Autodesk Inventor part; units mm, degrees
(part 4 of 18)
  ellipse E454 centre (-10072.3071, -10029.7963) end of major axis (-10072.1176, -10029.8098) minor radius 0.0836 (-10072.3568, -10029.8743) -> (-10072.2798, -10029.8808) ccw
  ellipse E455 centre (-10072.3658, -10028.6299) end of major axis (-10072.5466, -10028.6883) minor radius 0.168 (-10072.5392, -10028.5756) -> (-10072.5534, -10028.6311) ccw
  ellipse E456 centre (-10070.2632, -10029.6485) end of major axis (-10070.4527, -10029.6349) minor radius 0.0836 (-10070.2359, -10029.733) -> (-10070.1721, -10029.7273) ccw
  ellipse E457 centre (-10072.2975, -10029.6619) end of major axis (-10072.487, -10029.6483) minor radius 0.0836 (-10072.3473, -10029.7399) -> (-10072.2702, -10029.7464) ccw
  line L566 (-10072.7988, -10029.4384) -> (-10074.1814, -10029.4475)
  line L567 (-10074.3417, -10029.5333) -> (-10074.2688, -10029.759)
  line L568 (-10068.3003, -10029.8537) -> (-10068.4165, -10029.4942)
  line L569 (-10068.6314, -10029.4109) -> (-10070.0139, -10029.4201)
  line L570 (-10072.7892, -10029.3041) -> (-10074.1717, -10029.3132)
  line L571 (-10068.6218, -10029.2766) -> (-10070.0043, -10029.2857)
  line L572 (-10068.0936, -10030.3297) -> (-10068.4068, -10029.3599)
  ellipse E458 centre (-10074.1541, -10029.532) end of major axis (-10074.3436, -10029.5185) minor radius 0.0836 (-10074.1814, -10029.4475) -> (-10074.3417, -10029.5333) ccw
  ellipse E459 centre (-10068.6041, -10029.4955) end of major axis (-10068.4146, -10029.5091) minor radius 0.0836 (-10068.4165, -10029.4942) -> (-10068.6314, -10029.4109) ccw
  ellipse E460 centre (-10074.1444, -10029.3977) end of major axis (-10074.3339, -10029.3841) minor radius 0.0836 (-10074.1717, -10029.3132) -> (-10074.3339, -10029.3841) ccw
  ellipse E461 centre (-10068.5945, -10029.3611) end of major axis (-10068.4049, -10029.3747) minor radius 0.0836 (-10068.4068, -10029.3599) -> (-10068.6218, -10029.2766) ccw
  line L573 (-10074.3436, -10029.5185) -> (-10074.3339, -10029.3841)
  line L574 (-10068.0328, -10030.0942) -> (-10068.0416, -10030.217)
  line L575 (-10068.02, -10030.2837) -> (-10068.0042, -10030.0626)
  ellipse E462 centre (-10068.0775, -10030.1058) end of major axis (-10068.0759, -10030.3558) minor radius 0.0393 (-10068.0936, -10030.3297) -> (-10068.0416, -10030.217) ccw
  ellipse E463 centre (-10068.0775, -10030.1058) end of major axis (-10068.0802, -10029.7058) minor radius 0.0629 (-10068.0462, -10030.4607) -> (-10068.02, -10030.2837) ccw
  line L576 (-10072.5776, -10009.5324) -> (-10072.5771, -10009.4322)
  line L577 (-10072.56, -10009.5406) -> (-10072.5602, -10009.5699)
  line L578 (-10070.3424, -10009.4071) -> (-10072.3893, -10009.6071)
  ellipse E464 centre (-10074.1559, -10009.3828) end of major axis (-10074.3443, -10009.4073) minor radius 0.0925 (-10074.341, -10009.383) -> (-10074.3446, -10009.4012) ccw
  ellipse E465 centre (-10068.5548, -10008.9672) end of major axis (-10068.3664, -10008.9427) minor radius 0.0925 (-10068.366, -10008.9487) -> (-10068.3664, -10008.9427) ccw
  line L579 (-10068.3665, -10008.9422) -> (-10068.3664, -10008.9427)
  line L580 (-10074.3446, -10009.4012) -> (-10074.3449, -10009.4545)
  line L581 (-10068.3859, -10009.3883) -> (-10068.3843, -10009.0852)
  line L582 (-10068.3692, -10009.5702) -> (-10068.3673, -10009.1875)
  line L583 (-10068.366, -10008.9497) -> (-10068.366, -10008.9487)
  ellipse E466 centre (-10070.3419, -10009.314) end of major axis (-10070.1535, -10009.2894) minor radius 0.0925 (-10070.3424, -10009.4071) -> (-10070.1791, -10009.3449) ccw
  ellipse E467 centre (-10072.3888, -10009.5139) end of major axis (-10072.5772, -10009.5384) minor radius 0.0925 (-10072.5776, -10009.5324) -> (-10072.3893, -10009.6071) ccw
  line L584 (-10074.3428, -10028.4661) -> (-10074.3379, -10028.7031)
  line L585 (-10068.3814, -10029.0357) -> (-10068.3864, -10028.7937)
  line L586 (-10068.364, -10028.9277) -> (-10068.3693, -10028.6728)
  line L587 (-10072.5717, -10028.7608) -> (-10072.5745, -10028.6213)
  line L588 (-10071.9961, -10028.5946) -> (-10070.3406, -10028.7563)
  line L589 (-10072.5556, -10028.5861) -> (-10072.5548, -10028.6266)
  ellipse E468 centre (-10072.3858, -10028.6397) end of major axis (-10072.5743, -10028.616) minor radius 0.0827 (-10072.4425, -10028.5546) -> (-10072.5745, -10028.6213) ccw
  ellipse E469 centre (-10070.3389, -10028.8397) end of major axis (-10070.5274, -10028.816) minor radius 0.0827 (-10070.1715, -10028.8182) -> (-10070.3406, -10028.7563) ccw
  ellipse E470 centre (-10074.2929, -10028.3458) end of major axis (-10074.3318, -10028.7439) minor radius 0.023 (-10074.3379, -10028.7031) -> (-10074.3318, -10028.7439) ccw
  line L590 (-10074.3318, -10028.7439) -> (-10074.3186, -10028.7452)
  line L591 (-10068.0669, -10007.9159) -> (-10068.0533, -10008.0791)
  line L592 (-10068.0265, -10008.0749) -> (-10068.046, -10007.8415)
  ellipse E471 centre (-10068.2546, -10007.9147) end of major axis (-10068.0717, -10007.9662) minor radius 0.1628 (-10068.0669, -10007.9159) -> (-10068.1028, -10007.8283) ccw
  ellipse E472 centre (-10068.2336, -10007.8402) end of major axis (-10068.0507, -10007.8917) minor radius 0.1628 (-10068.046, -10007.8415) -> (-10068.0637, -10007.7817) ccw
  line L593 (-10072.5692, -10008.6941) -> (-10072.5188, -10008.5152)
  line L594 (-10072.274, -10008.3132) -> (-10070.2397, -10008.3266)
  ellipse E473 centre (-10072.5402, -10009.0414) end of major axis (-10072.5376, -10008.6414) minor radius 0.0629 (-10072.5692, -10008.6941) -> (-10072.5961, -10009.2399) ccw
  line L595 (-10072.5794, -10009.4405) -> (-10072.5961, -10009.2399)
  line L596 (-10072.5752, -10009.1654) -> (-10072.5402, -10009.5845)
  ellipse E474 centre (-10072.5402, -10009.0414) end of major axis (-10072.5419, -10009.2914) minor radius 0.0393 (-10072.5584, -10008.8243) -> (-10072.5752, -10009.1654) ccw
  line L597 (-10072.5129, -10008.6627) -> (-10072.5584, -10008.8243)
  line L598 (-10070.1865, -10009.2558) -> (-10070.1769, -10009.3706)
  ellipse E475 centre (-10070.1306, -10009.0573) end of major axis (-10070.1333, -10009.4572) minor radius 0.0629 (-10070.169, -10008.7504) -> (-10070.1865, -10009.2558) ccw
  line L599 (-10070.2288, -10008.4569) -> (-10070.6802, -10008.4539)
  line L600 (-10071.7883, -10008.4466) -> (-10072.2631, -10008.4435)
  ellipse E476 centre (-10072.3006, -10008.4075) end of major axis (-10072.4899, -10008.4233) minor radius 0.0933 (-10072.274, -10008.3132) -> (-10072.3541, -10008.3212) ccw
  ellipse E477 centre (-10070.2662, -10008.4209) end of major axis (-10070.4556, -10008.4367) minor radius 0.0933 (-10070.139, -10008.3436) -> (-10070.2397, -10008.3266) ccw
  ellipse E478 centre (-10072.2897, -10008.5377) end of major axis (-10072.1003, -10008.5219) minor radius 0.0933 (-10072.2631, -10008.4435) -> (-10072.3224, -10008.4477) ccw
  ellipse E479 centre (-10070.2554, -10008.5511) end of major axis (-10070.066, -10008.5353) minor radius 0.0933 (-10070.2169, -10008.4571) -> (-10070.2288, -10008.4569) ccw
  ellipse E480 centre (-10070.2554, -10008.5511) end of major axis (-10070.066, -10008.5353) minor radius 0.0933 (-10070.1515, -10008.4664) -> (-10070.1951, -10008.4587) ccw
  line L601 (-10068.4018, -10008.7216) -> (-10068.3587, -10008.5683)
  line L602 (-10068.3909, -10008.8518) -> (-10068.0864, -10007.77)
  line L603 (-10074.3539, -10009.2283) -> (-10074.3358, -10009.4456)
  ellipse E481 centre (-10068.3728, -10009.0688) end of major axis (-10068.3712, -10008.8188) minor radius 0.0393 (-10068.3909, -10008.8518) -> (-10068.4083, -10009.1858) ccw
  ellipse E482 centre (-10074.2981, -10009.0298) end of major axis (-10074.3007, -10009.4298) minor radius 0.0629 (-10074.3322, -10008.7027) -> (-10074.3539, -10009.2283) ccw
  ellipse E483 centre (-10068.3728, -10009.0688) end of major axis (-10068.3755, -10009.4688) minor radius 0.0629 (-10068.4018, -10008.7216) -> (-10068.4291, -10009.2632) ccw
  ellipse E484 centre (-10068.274, -10007.7687) end of major axis (-10068.0847, -10007.7529) minor radius 0.0933 (-10068.0864, -10007.77) -> (-10068.0847, -10007.7529) ccw
  line L604 (-10068.0891, -10007.6998) -> (-10068.0847, -10007.7529)
  ellipse E485 centre (-10068.2166, -10029.1254) end of major axis (-10068.2055, -10029.5678) minor radius 0.0741 (-10068.2815, -10029.2883) -> (-10068.2747, -10029.3519) ccw
  ellipse E486 centre (-10068.255, -10029.2752) end of major axis (-10068.2588, -10029.1252) minor radius 0.0251 (-10068.2747, -10029.3519) -> (-10068.2615, -10029.4132) ccw
  ellipse E487 centre (-10068.0941, -10029.6595) end of major axis (-10068.0903, -10029.8095) minor radius 0.0251 (-10068.1005, -10029.7976) -> (-10068.0913, -10029.8094) ccw
  ellipse E488 centre (-10068.081, -10029.626) end of major axis (-10068.0772, -10029.7759) minor radius 0.0251 (-10068.0646, -10029.7534) -> (-10068.0639, -10029.7505) ccw
  line L605 (-10068.1005, -10029.7976) -> (-10068.1215, -10029.7476)
  line L606 (-10068.1648, -10029.6441) -> (-10068.1786, -10029.611)
  line L607 (-10068.2503, -10029.4398) -> (-10068.2615, -10029.4132)
  line L608 (-10068.176, -10028.1752) -> (-10068.1513, -10028.2344)
  ellipse E489 centre (-10068.1507, -10028.9567) end of major axis (-10068.1653, -10028.3769) minor radius 0.0971 (-10068.2473, -10028.9755) -> (-10068.1981, -10029.4188) ccw
  ellipse E490 centre (-10068.2342, -10029.4508) end of major axis (-10068.2418, -10029.3009) minor radius 0.0268 (-10068.2599, -10029.4689) -> (-10068.2591, -10029.4803) ccw
  ellipse E491 centre (-10068.2342, -10029.4508) end of major axis (-10068.2418, -10029.3009) minor radius 0.0268 (-10068.262, -10029.415) -> (-10068.2619, -10029.4249) ccw
  ellipse E492 centre (-10068.2245, -10029.5349) end of major axis (-10068.2321, -10029.3851) minor radius 0.0268 (-10068.2444, -10029.6076) -> (-10068.2291, -10029.6709) ccw
  ellipse E493 centre (-10068.0447, -10029.9467) end of major axis (-10068.0371, -10030.0965) minor radius 0.0268 (-10068.0493, -10030.0827) -> (-10068.0322, -10030.0935) ccw
  ellipse E494 centre (-10068.0311, -10029.9157) end of major axis (-10068.0235, -10030.0655) minor radius 0.0268 (-10068.0117, -10030.0467) -> (-10068.0037, -10029.9785) ccw
  line L609 (-10068.051, -10030.0972) -> (-10068.0371, -10030.0965)
  ellipse E495 centre (-10068.1857, -10029.3931) end of major axis (-10068.1633, -10029.8351) minor radius 0.0791 (-10068.2591, -10029.4803) -> (-10068.2444, -10029.6076) ccw
  ellipse E496 centre (-10068.069, -10029.6603) end of major axis (-10068.0467, -10030.1022) minor radius 0.0791 (-10068.0322, -10030.0935) -> (-10068.0117, -10030.0467) ccw
  line L610 (-10068.0493, -10030.0827) -> (-10068.2291, -10029.6709)
  line L611 (-10067.9958, -10029.7471) -> (-10068.0037, -10029.9785)
  ellipse E497 centre (-10068.1176, -10029.2376) end of major axis (-10068.0883, -10029.8168) minor radius 0.1037 (-10068.2225, -10029.2114) -> (-10068.0439, -10029.7495) ccw
  ellipse E498 centre (-10068.0426, -10008.2513) end of major axis (-10068.0502, -10008.4011) minor radius 0.0268 (-10068.0158, -10008.1748) -> (-10068.0253, -10008.1135) ccw
  ellipse E499 centre (-10068.0571, -10008.2291) end of major axis (-10068.0495, -10008.0793) minor radius 0.0268 (-10068.0472, -10008.08) -> (-10068.0645, -10008.1003) ccw
  ellipse E500 centre (-10068.2329, -10008.7305) end of major axis (-10068.2253, -10008.5807) minor radius 0.0268 (-10068.2403, -10008.6017) -> (-10068.2547, -10008.6717) ccw
  ellipse E501 centre (-10068.2411, -10008.8174) end of major axis (-10068.2335, -10008.6676) minor radius 0.0268 (-10068.2683, -10008.8855) -> (-10068.2679, -10008.8939) ccw
  line L612 (-10068.0495, -10008.0793) -> (-10068.0671, -10008.0784)
  ellipse E502 centre (-10068.0763, -10008.5199) end of major axis (-10068.0539, -10008.078) minor radius 0.0791 (-10068.0253, -10008.1135) -> (-10068.0472, -10008.08) ccw
  ellipse E503 centre (-10068.1903, -10008.8452) end of major axis (-10068.2127, -10009.2872) minor radius 0.0791 (-10068.2547, -10008.6717) -> (-10068.2605, -10008.7235) ccw
  line L613 (-10068.2403, -10008.6017) -> (-10068.0645, -10008.1003)
  line L614 (-10068.2516, -10009.1768) -> (-10068.2518, -10009.1737)
  line L615 (-10068.2642, -10008.9583) -> (-10068.2679, -10008.8939)
  line L616 (-10068.0158, -10008.1748) -> (-10068.0001, -10008.4467)
  ellipse E504 centre (-10068.1176, -10008.9564) end of major axis (-10068.0883, -10008.3771) minor radius 0.1037 (-10068.0439, -10008.4445) -> (-10068.2225, -10008.9826) ccw
  line L617 (-10068.0719, -10010.0812) -> (-10068.0313, -10009.9604)
  ellipse E505 centre (-10067.8862, -10010.5697) end of major axis (-10067.942, -10009.9924) minor radius 0.1485 (-10067.9286, -10009.9934) -> (-10068.0078, -10010.0749) ccw
  line L618 (-10068.0318, -10028.2336) -> (-10068.0835, -10028.1117)
  ellipse E506 centre (-10067.8862, -10027.6243) end of major axis (-10067.942, -10028.2016) minor radius 0.1485 (-10068.0078, -10028.1191) -> (-10067.9286, -10028.2006) ccw
  ellipse E507 centre (-10068.2842, -10028.9429) end of major axis (-10068.2852, -10028.7929) minor radius 0.0236 (-10068.3057, -10028.8761) -> (-10068.3073, -10028.9683) ccw
  ellipse E508 centre (-10068.2791, -10029.028) end of major axis (-10068.2801, -10028.878) minor radius 0.0236 (-10068.2996, -10029.097) -> (-10068.2888, -10029.1623) ccw
  ellipse E509 centre (-10068.2392, -10028.8933) end of major axis (-10068.2363, -10029.3358) minor radius 0.0696 (-10068.3073, -10028.9683) -> (-10068.2996, -10029.097) ccw
  line L619 (-10068.2662, -10029.2321) -> (-10068.2888, -10029.1623)
  line L620 (-10068.1312, -10028.107) -> (-10068.0902, -10028.234)
  line L621 (-10068.3057, -10028.8761) -> (-10068.2498, -10028.0954)
  ellipse E510 centre (-10068.1729, -10028.7496) end of major axis (-10068.1767, -10028.1696) minor radius 0.0912 (-10068.1343, -10028.2343) -> (-10068.2194, -10029.236) ccw
  ellipse E511 centre (-10068.2956, -10009.9174) end of major axis (-10068.2811, -10010.0667) minor radius 0.0086 (-10068.3042, -10009.7865) -> (-10068.3053, -10009.7814) ccw
  ellipse E512 centre (-10068.2956, -10009.9174) end of major axis (-10068.2811, -10010.0667) minor radius 0.0086 (-10068.2953, -10009.8439) -> (-10068.2956, -10009.8416) ccw
  ellipse E513 centre (-10068.303, -10009.8935) end of major axis (-10068.3175, -10009.7442) minor radius 0.0086 (-10068.3164, -10009.7453) -> (-10068.3199, -10009.7636) ccw
  line L622 (-10068.3175, -10009.7442) -> (-10068.345, -10009.7469)
  ellipse E514 centre (-10068.2768, -10010.1827) end of major axis (-10068.3198, -10009.7423) minor radius 0.0254 (-10068.3053, -10009.7814) -> (-10068.3164, -10009.7453) ccw
  line L623 (-10068.3219, -10010.1562) -> (-10068.3199, -10009.7636)
  line L624 (-10068.2953, -10009.8439) -> (-10068.2619, -10010.0997)
  ellipse E515 centre (-10068.2416, -10010.6152) end of major axis (-10068.298, -10010.038) minor radius 0.0333 (-10068.2764, -10010.1012) -> (-10068.3066, -10010.1585) ccw
  line L625 (-10068.3164, -10028.4243) -> (-10068.3244, -10028.0381)
  line L626 (-10068.2611, -10028.0943) -> (-10068.2905, -10028.3273)
  ellipse E516 centre (-10068.2995, -10028.2903) end of major axis (-10068.3141, -10028.4396) minor radius 0.0086 (-10068.3164, -10028.4243) -> (-10068.3124, -10028.4373) ccw
  ellipse E517 centre (-10068.2918, -10028.2614) end of major axis (-10068.3064, -10028.4107) minor radius 0.0086 (-10068.3007, -10028.3936) -> (-10068.2905, -10028.3273) ccw
  line L627 (-10068.3314, -10028.4379) -> (-10068.3141, -10028.4396)
  ellipse E518 centre (-10068.2746, -10028.0036) end of major axis (-10068.3176, -10028.444) minor radius 0.0254 (-10068.3124, -10028.4373) -> (-10068.3007, -10028.3936) ccw
  ellipse E519 centre (-10068.2416, -10027.5788) end of major axis (-10068.298, -10028.156) minor radius 0.0333 (-10068.3066, -10028.0354) -> (-10068.2764, -10028.0928) ccw
  line L628 (-10068.2926, -10009.0763) -> (-10068.2428, -10008.8992)
  line L629 (-10068.2069, -10008.7717) -> (-10068.2045, -10008.7632)
  line L630 (-10068.246, -10010.0982) -> (-10068.307, -10009.3676)
  line L631 (-10068.0946, -10009.9599) -> (-10068.1304, -10010.0869)
  ellipse E520 centre (-10068.2818, -10009.2065) end of major axis (-10068.2808, -10009.0565) minor radius 0.0236 (-10068.2926, -10009.0763) -> (-10068.3029, -10009.1453) ccw
  ellipse E521 centre (-10068.286, -10009.2931) end of major axis (-10068.2851, -10009.1431) minor radius 0.0236 (-10068.3094, -10009.2764) -> (-10068.307, -10009.3676) ccw
  ellipse E522 centre (-10068.2405, -10009.3258) end of major axis (-10068.2435, -10009.7683) minor radius 0.0696 (-10068.3029, -10009.1453) -> (-10068.3094, -10009.2764) ccw
  ellipse E523 centre (-10068.1729, -10009.4444) end of major axis (-10068.1767, -10010.0244) minor radius 0.0912 (-10068.2194, -10008.9579) -> (-10068.1343, -10009.9597) ccw
  line L632 (-10070.1822, -10029.6789) -> (-10070.1714, -10029.7049)
  line L633 (-10072.2585, -10029.7464) -> (-10072.2648, -10029.7314)
  line L634 (-10070.1801, -10029.6329) -> (-10070.1698, -10029.6576)
  line L635 (-10070.1822, -10029.6789) -> (-10070.2823, -10029.6815)
  ellipse E524 centre (-10070.3232, -10029.5837) end of major axis (-10070.5729, -10029.572) minor radius 0.0974 (-10070.5696, -10029.5899) -> (-10070.2823, -10029.6815) ccw
  line L636 (-10070.5696, -10029.5899) -> (-10070.716, -10029.2401)
  line L637 (-10070.831, -10029.2035) -> (-10072.0235, -10029.2335)
  line L638 (-10072.1057, -10029.2751) -> (-10072.013, -10029.4965)
  ellipse E525 centre (-10072.2056, -10029.6311) end of major axis (-10072.4554, -10029.6195) minor radius 0.0974 (-10072.1647, -10029.7289) -> (-10072.0301, -10029.7074) ccw
  line L639 (-10072.1647, -10029.7289) -> (-10072.2648, -10029.7314)
  line L640 (-10072.0214, -10029.1875) -> (-10070.8288, -10029.1575)
  line L641 (-10072.2626, -10029.6854) -> (-10072.1626, -10029.6829)
  ellipse E526 centre (-10072.2035, -10029.5851) end of major axis (-10071.9538, -10029.5968) minor radius 0.0974 (-10072.1626, -10029.6829) -> (-10072.0476, -10029.6675) ccw
  line L642 (-10070.7139, -10029.1941) -> (-10070.5674, -10029.5439)
  ellipse E527 centre (-10070.321, -10029.5377) end of major axis (-10070.5708, -10029.526) minor radius 0.0974 (-10070.5674, -10029.5439) -> (-10070.2801, -10029.6355) ccw
  line L643 (-10070.2801, -10029.6355) -> (-10070.1801, -10029.6329)
  line L644 (-10072.2648, -10029.7314) -> (-10072.2626, -10029.6854)
  line L645 (-10070.1801, -10029.6329) -> (-10070.1822, -10029.6789)
  ellipse E528 centre (-10070.8146, -10029.2426) end of major axis (-10070.7147, -10029.2472) minor radius 0.0389 (-10070.716, -10029.2401) -> (-10070.831, -10029.2035) ccw
  ellipse E529 centre (-10072.0071, -10029.2726) end of major axis (-10072.107, -10029.268) minor radius 0.0389 (-10072.0235, -10029.2335) -> (-10072.1057, -10029.2751) ccw
  ellipse E530 centre (-10070.8124, -10029.1966) end of major axis (-10070.7125, -10029.2012) minor radius 0.0389 (-10070.7139, -10029.1941) -> (-10070.8288, -10029.1575) ccw
  ellipse E531 centre (-10072.005, -10029.2266) end of major axis (-10072.1049, -10029.2219) minor radius 0.0389 (-10072.0214, -10029.1875) -> (-10072.1049, -10029.2219) ccw
  line L646 (-10072.107, -10029.268) -> (-10072.1049, -10029.2219)
  line L647 (-10070.2419, -10009.1799) -> (-10070.2377, -10009.2298)
  line L648 (-10072.3244, -10009.1274) -> (-10072.3222, -10009.1544)
  line L649 (-10070.2283, -10009.2232) -> (-10070.2342, -10009.1527)
  ellipse E532 centre (-10070.5084, -10008.9693) end of major axis (-10070.7489, -10008.9011) minor radius 0.2063 (-10070.5471, -10009.1722) -> (-10070.4354, -10009.175) ccw
  ellipse E533 centre (-10072.0922, -10008.9293) end of major axis (-10072.3328, -10008.8612) minor radius 0.2063 (-10072.1309, -10009.1323) -> (-10072.0193, -10009.1351) ccw
  spline S14 degree 3 poles (-10070.5156, -10008.7469) (-10070.5214, -10008.7475) (-10070.533, -10008.7488) (-10070.5501, -10008.752) (-10070.5668, -10008.7561) (-10070.583, -10008.7613) (-10070.5987, -10008.7673) (-10070.6139, -10008.7742) (-10070.6284, -10008.782) (-10070.6421, -10008.7906) (-10070.6552, -10008.7999) (-10070.6674, -10008.8099) (-10070.6787, -10008.8207) (-10070.6891, -10008.8321) (-10070.6985, -10008.8441) (-10070.7068, -10008.8567) (-10070.7141, -10008.8698) (-10070.7179, -10008.879) (-10070.7199, -10008.8836) knots 0 0 0 0 0.068015 0.135329 0.201939 0.267833 0.332993 0.397396 0.46102 0.523846 0.585863 0.647073 0.70749 0.767154 0.826125 0.884497 0.9424 1 1 1 1
  spline S15 degree 3 poles (-10070.713, -10009.0173) (-10070.7109, -10009.0213) (-10070.7069, -10009.0293) (-10070.6998, -10009.0408) (-10070.6919, -10009.0518) (-10070.6834, -10009.0624) (-10070.6741, -10009.0725) (-10070.6642, -10009.0821) (-10070.6538, -10009.0911) (-10070.6427, -10009.0996) (-10070.6312, -10009.1076) (-10070.6191, -10009.1149) (-10070.6067, -10009.1216) (-10070.5938, -10009.1277) (-10070.5806, -10009.1331) (-10070.5671, -10009.1378) (-10070.5534, -10009.1419) (-10070.5441, -10009.144) (-10070.5394, -10009.145) knots 0 0 0 0 0.060188 0.120572 0.181231 0.242221 0.303577 0.365317 0.427444 0.489947 0.552805 0.61599 0.67947 0.743206 0.807162 0.871301 0.93559 1 1 1 1
  spline S16 degree 3 poles (-10070.5471, -10009.1722) (-10070.5517, -10009.171) (-10070.5609, -10009.1686) (-10070.5744, -10009.1638) (-10070.5876, -10009.1581) (-10070.6004, -10009.1515) (-10070.6128, -10009.1441) (-10070.6249, -10009.1359) (-10070.6365, -10009.127) (-10070.6476, -10009.1174) (-10070.6582, -10009.1071) (-10070.6684, -10009.0963) (-10070.6779, -10009.0848) (-10070.6869, -10009.0729) (-10070.6952, -10009.0605) (-10070.703, -10009.0476) (-10070.71, -10009.0345) (-10070.7142, -10009.0254) (-10070.7162, -10009.0208) knots 0 0 0 0 0.060752 0.121577 0.182585 0.243852 0.305433 0.367353 0.42962 0.492223 0.555134 0.618315 0.681718 0.745286 0.808961 0.872679 0.936378 1 1 1 1
  spline S17 degree 3 poles (-10070.7384, -10008.9155) (-10070.7381, -10008.9083) (-10070.7374, -10008.8939) (-10070.7337, -10008.8724) (-10070.7279, -10008.8517) (-10070.7199, -10008.832) (-10070.71, -10008.8137) (-10070.6984, -10008.7968) (-10070.6853, -10008.7813) (-10070.6707, -10008.7672) (-10070.6548, -10008.7545) (-10070.6377, -10008.7433) (-10070.6197, -10008.7334) (-10070.6008, -10008.7249) (-10070.5811, -10008.7178) (-10070.5608, -10008.7121) (-10070.5401, -10008.7076) (-10070.5261, -10008.7058) (-10070.5191, -10008.7049) knots 0 0 0 0 0.06487 0.129748 0.194733 0.25818 0.320168 0.381236 0.441837 0.502335 0.563004 0.624034 0.685537 0.747559 0.810091 0.873076 0.936419 1 1 1 1
  spline S18 degree 3 poles (-10070.407, -10008.7077) (-10070.4007, -10008.709) (-10070.3884, -10008.7114) (-10070.3706, -10008.7172) (-10070.3538, -10008.7245) (-10070.3381, -10008.7332) (-10070.3235, -10008.7432) (-10070.3101, -10008.7546) (-10070.2978, -10008.7672) (-10070.2868, -10008.781) (-10070.277, -10008.7959) (-10070.2685, -10008.8119) (-10070.2613, -10008.8287) (-10070.2555, -10008.8465) (-10070.2511, -10008.8651) (-10070.2481, -10008.8845) (-10070.2466, -10008.9045) (-10070.2468, -10008.9181) (-10070.2469, -10008.9249) knots 0 0 0 0 0.064651 0.127488 0.188893 0.249239 0.308882 0.368162 0.427398 0.486884 0.546892 0.60767 0.669446 0.732427 0.796802 0.862747 0.930428 1 1 1 1
  spline S19 degree 3 poles (-10070.2695, -10009.0294) (-10070.2715, -10009.0341) (-10070.2755, -10009.0434) (-10070.2824, -10009.0569) (-10070.2899, -10009.0698) (-10070.2981, -10009.0822) (-10070.3068, -10009.0939) (-10070.3161, -10009.1051) (-10070.3259, -10009.1155) (-10070.3363, -10009.1253) (-10070.3471, -10009.1344) (-10070.3585, -10009.1427) (-10070.3703, -10009.1503) (-10070.3826, -10009.157) (-10070.3952, -10009.1629) (-10070.4083, -10009.1679) (-10070.4217, -10009.172) (-10070.4308, -10009.174) (-10070.4354, -10009.175) knots 0 0 0 0 0.066474 0.132184 0.19716 0.261439 0.325059 0.388062 0.450498 0.512425 0.573908 0.635026 0.695866 0.756532 0.81714 0.87782 0.938719 1 1 1 1
  spline S20 degree 3 poles (-10070.4277, -10009.1478) (-10070.4243, -10009.1472) (-10070.4174, -10009.146) (-10070.4073, -10009.1435) (-10070.3973, -10009.1405) (-10070.3876, -10009.1371) (-10070.3782, -10009.1332) (-10070.3659, -10009.1273) (-10070.3511, -10009.119) (-10070.3344, -10009.1074) (-10070.3189, -10009.0944) (-10070.3044, -10009.0802) (-10070.2959, -10009.0698) (-10070.2916, -10009.0646) knots 0 0 0 0 0.064451 0.128324 0.191723 0.254738 0.31745 0.379928 0.504372 0.628458 0.752389 0.876245 1 1 1 1
  spline S21 degree 3 poles (-10070.2513, -10008.8502) (-10070.2528, -10008.8468) (-10070.2559, -10008.8398) (-10070.2616, -10008.83) (-10070.2679, -10008.8207) (-10070.2749, -10008.812) (-10070.2826, -10008.8039) (-10070.2909, -10008.7962) (-10070.2998, -10008.7891) (-10070.3093, -10008.7826) (-10070.3194, -10008.7766) (-10070.33, -10008.7712) (-10070.3411, -10008.7662) (-10070.3527, -10008.7619) (-10070.3648, -10008.758) (-10070.3773, -10008.7547) (-10070.3902, -10008.7518) (-10070.399, -10008.7504) (-10070.4035, -10008.7497) knots 0 0 0 0 0.059947 0.119085 0.177737 0.236204 0.294771 0.353693 0.413202 0.473501 0.534763 0.597137 0.660745 0.725684 0.792031 0.859842 0.929157 1 1 1 1
  spline S22 degree 3 poles (-10072.0994, -10008.707) (-10072.1058, -10008.7077) (-10072.1185, -10008.7091) (-10072.1373, -10008.7128) (-10072.1556, -10008.7177) (-10072.1733, -10008.7237) (-10072.1903, -10008.7308) (-10072.2066, -10008.7389) (-10072.222, -10008.748) (-10072.2366, -10008.7581) (-10072.2502, -10008.7691) (-10072.2627, -10008.7809) (-10072.2741, -10008.7935) (-10072.2842, -10008.8068) (-10072.2931, -10008.8208) (-10072.3005, -10008.8355) (-10072.3066, -10008.8508) (-10072.3094, -10008.8614) (-10072.3107, -10008.8666) knots 0 0 0 0 0.068478 0.136179 0.203098 0.269216 0.33451 0.398951 0.462515 0.525184 0.586956 0.647848 0.707903 0.767201 0.825862 0.884056 0.942007 1 1 1 1
  spline S23 degree 3 poles (-10072.2881, -10008.9935) (-10072.2859, -10008.997) (-10072.2815, -10009.004) (-10072.2741, -10009.014) (-10072.2662, -10009.0236) (-10072.2577, -10009.0328) (-10072.2487, -10009.0416) (-10072.2392, -10009.0499) (-10072.2292, -10009.0578) (-10072.2187, -10009.0652) (-10072.2079, -10009.0721) (-10072.1966, -10009.0785) (-10072.1851, -10009.0844) (-10072.1732, -10009.0897) (-10072.161, -10009.0945) (-10072.1486, -10009.0987) (-10072.136, -10009.1023) (-10072.1275, -10009.1042) (-10072.1232, -10009.1051) knots 0 0 0 0 0.06026 0.120787 0.181623 0.242797 0.30432 0.366196 0.428417 0.490967 0.553825 0.616963 0.680352 0.743961 0.807759 0.871715 0.935803 1 1 1 1
  spline S24 degree 3 poles (-10072.1309, -10009.1323) (-10072.1352, -10009.1312) (-10072.1437, -10009.129) (-10072.1563, -10009.1246) (-10072.1685, -10009.1195) (-10072.1805, -10009.1136) (-10072.1922, -10009.107) (-10072.2035, -10009.0996) (-10072.2145, -10009.0917) (-10072.225, -10009.0831) (-10072.2352, -10009.0739) (-10072.2449, -10009.0642) (-10072.2542, -10009.054) (-10072.263, -10009.0433) (-10072.2712, -10009.0322) (-10072.279, -10009.0207) (-10072.2862, -10009.0088) (-10072.2905, -10009.0006) (-10072.2927, -10008.9965) knots 0 0 0 0 0.060837 0.121734 0.182787 0.244069 0.305631 0.367501 0.429693 0.492205 0.555019 0.618108 0.681437 0.744961 0.808632 0.872398 0.936205 1 1 1 1
  spline S25 degree 3 poles (-10072.3215, -10008.8966) (-10072.3219, -10008.889) (-10072.3226, -10008.8736) (-10072.3208, -10008.8506) (-10072.3165, -10008.828) (-10072.3097, -10008.8062) (-10072.3006, -10008.7858) (-10072.2895, -10008.7669) (-10072.2765, -10008.7496) (-10072.2618, -10008.7339) (-10072.2455, -10008.7198) (-10072.2279, -10008.7073) (-10072.2091, -10008.6963) (-10072.1892, -10008.6869) (-10072.1685, -10008.6791) (-10072.1471, -10008.6728) (-10072.1252, -10008.6679) (-10072.1104, -10008.666) (-10072.1029, -10008.665) knots 0 0 0 0 0.064914 0.129619 0.19438 0.258975 0.321768 0.383219 0.443897 0.504267 0.56469 0.625418 0.686613 0.748349 0.81063 0.873405 0.936573 1 1 1 1
  spline S26 degree 3 poles (-10071.9908, -10008.6678) (-10071.9842, -10008.6692) (-10071.9712, -10008.6718) (-10071.9525, -10008.678) (-10071.9349, -10008.6859) (-10071.9186, -10008.6954) (-10071.9034, -10008.7064) (-10071.8896, -10008.7188) (-10071.8771, -10008.7326) (-10071.866, -10008.7477) (-10071.8563, -10008.764) (-10071.848, -10008.7814) (-10071.8413, -10008.7998) (-10071.8361, -10008.8192) (-10071.8326, -10008.8394) (-10071.8306, -10008.8604) (-10071.8303, -10008.8821) (-10071.8315, -10008.8967) (-10071.8321, -10008.9042) knots 0 0 0 0 0.064101 0.126323 0.187089 0.246808 0.305872 0.364653 0.423494 0.482714 0.542601 0.60342 0.665411 0.728789 0.793757 0.860499 0.92919 1 1 1 1
  spline S27 degree 3 poles (-10071.8619, -10009.0082) (-10071.864, -10009.0123) (-10071.8682, -10009.0204) (-10071.8752, -10009.0321) (-10071.8827, -10009.0434) (-10071.8907, -10009.0541) (-10071.8992, -10009.0644) (-10071.9082, -10009.074) (-10071.9176, -10009.0831) (-10071.9274, -10009.0916) (-10071.9376, -10009.0995) (-10071.9482, -10009.1067) (-10071.9592, -10009.1133) (-10071.9706, -10009.1191) (-10071.9823, -10009.1243) (-10071.9943, -10009.1287) (-10072.0066, -10009.1324) (-10072.015, -10009.1342) (-10072.0193, -10009.1351) knots 0 0 0 0 0.065853 0.13104 0.19559 0.259537 0.322916 0.38577 0.448145 0.510097 0.571687 0.632987 0.694078 0.755051 0.81601 0.877068 0.938352 1 1 1 1
  spline S28 degree 3 poles (-10072.0116, -10009.1079) (-10072.0081, -10009.1073) (-10072.0012, -10009.1061) (-10071.9911, -10009.1036) (-10071.9811, -10009.1006) (-10071.9714, -10009.0972) (-10071.962, -10009.0932) (-10071.9497, -10009.0874) (-10071.9349, -10009.0791) (-10071.9182, -10009.0675) (-10071.9027, -10009.0545) (-10071.8883, -10009.0403) (-10071.8797, -10009.0299) (-10071.8754, -10009.0247) knots 0 0 0 0 0.064451 0.128324 0.191723 0.254738 0.31745 0.379928 0.504372 0.628458 0.752389 0.876245 1 1 1 1
  spline S29 degree 3 poles (-10071.8351, -10008.8103) (-10071.8367, -10008.8069) (-10071.8398, -10008.7999) (-10071.8454, -10008.7901) (-10071.8517, -10008.7808) (-10071.8588, -10008.7721) (-10071.8664, -10008.7639) (-10071.8747, -10008.7563) (-10071.8836, -10008.7492) (-10071.8931, -10008.7427) (-10071.9032, -10008.7367) (-10071.9138, -10008.7313) (-10071.9249, -10008.7263) (-10071.9365, -10008.7219) (-10071.9486, -10008.7181) (-10071.9611, -10008.7148) (-10071.9741, -10008.7119) (-10071.9829, -10008.7105) (-10071.9873, -10008.7098) knots 0 0 0 0 0.059947 0.119085 0.177737 0.236204 0.294771 0.353693 0.413202 0.473501 0.534763 0.597137 0.660745 0.725684 0.792031 0.859842 0.929157 1 1 1 1
  ellipse E534 centre (-10070.5005, -10008.8386) end of major axis (-10070.2514, -10008.8177) minor radius 0.1348 (-10070.407, -10008.7077) -> (-10070.5191, -10008.7049) ccw
  ellipse E535 centre (-10070.497, -10008.8805) end of major axis (-10070.7461, -10008.9015) minor radius 0.1348 (-10070.4035, -10008.7497) -> (-10070.5156, -10008.7469) ccw
  ellipse E536 centre (-10072.0843, -10008.7987) end of major axis (-10071.8352, -10008.7778) minor radius 0.1348 (-10071.9908, -10008.6678) -> (-10072.1029, -10008.665) ccw
  ellipse E537 centre (-10072.0808, -10008.8406) end of major axis (-10072.3299, -10008.8615) minor radius 0.1348 (-10071.9873, -10008.7098) -> (-10072.0994, -10008.707) ccw
  ellipse E538 centre (-10070.5007, -10008.9421) end of major axis (-10070.2602, -10009.0102) minor radius 0.2063 (-10070.5394, -10009.145) -> (-10070.4277, -10009.1478) ccw
  ellipse E539 centre (-10072.0845, -10008.9022) end of major axis (-10071.844, -10008.9703) minor radius 0.2063 (-10072.1232, -10009.1051) -> (-10072.0116, -10009.1079) ccw
  ellipse E540 centre (-10070.1899, -10008.9962) end of major axis (-10070.1826, -10008.7083) minor radius 0.0482 (-10070.2376, -10008.9791) -> (-10070.2342, -10009.1527) ccw
  ellipse E541 centre (-10070.1899, -10008.9962) end of major axis (-10070.1826, -10008.7083) minor radius 0.0482 (-10070.2102, -10008.7546) -> (-10070.2314, -10008.8822) ccw
  ellipse E542 centre (-10070.1899, -10008.9962) end of major axis (-10070.1984, -10009.3341) minor radius 0.0566 (-10070.2137, -10008.7126) -> (-10070.2434, -10008.9231) ccw
  ellipse E543 centre (-10070.1899, -10008.9962) end of major axis (-10070.1984, -10009.3341) minor radius 0.0566 (-10070.2471, -10009.0515) -> (-10070.2419, -10009.1799) ccw
  ellipse E544 centre (-10072.2724, -10008.9438) end of major axis (-10072.2809, -10009.2817) minor radius 0.0566 (-10072.2962, -10008.6601) -> (-10072.3284, -10008.9233) ccw
  ellipse E545 centre (-10072.2724, -10008.9438) end of major axis (-10072.2809, -10009.2817) minor radius 0.0566 (-10072.3284, -10009.0611) -> (-10072.3244, -10009.1274) ccw
  line L650 (-10070.1537, -10008.5006) -> (-10070.2137, -10008.7126)
  line L651 (-10072.2962, -10008.6601) -> (-10072.2875, -10008.6294)
  line L652 (-10072.2626, -10008.5413) -> (-10072.2349, -10008.4436)
  line L653 (-10070.1563, -10008.5644) -> (-10070.2102, -10008.7546)
  line L654 (-10070.5546, -10029.8434) -> (-10070.6969, -10029.5177)
  line L655 (-10070.8135, -10029.4808) -> (-10072.0025, -10029.5409)
  line L656 (-10072.0824, -10029.5877) -> (-10071.9188, -10029.9624)
  ellipse E546 centre (-10072.1644, -10029.9749) end of major axis (-10071.9146, -10029.9833) minor radius 0.1052 (-10072.059, -10030.0732) -> (-10071.9188, -10029.9624) ccw
  line L657 (-10072.0009, -10029.4955) -> (-10070.8119, -10029.4354)
  line L658 (-10070.6954, -10029.4723) -> (-10070.5528, -10029.7986)
  line L659 (-10072.2182, -10030.0772) -> (-10072.2181, -10030.0742)
  ellipse E547 centre (-10070.7952, -10029.5226) end of major axis (-10070.6952, -10029.526) minor radius 0.0421 (-10070.6969, -10029.5177) -> (-10070.8135, -10029.4808) ccw
  ellipse E548 centre (-10071.9842, -10029.5828) end of major axis (-10072.0841, -10029.5794) minor radius 0.0421 (-10072.0025, -10029.5409) -> (-10072.0824, -10029.5877) ccw
  ellipse E549 centre (-10070.7936, -10029.4773) end of major axis (-10070.6937, -10029.4807) minor radius 0.0421 (-10070.6954, -10029.4723) -> (-10070.8119, -10029.4354) ccw
  ellipse E550 centre (-10071.9826, -10029.5374) end of major axis (-10072.0826, -10029.534) minor radius 0.0421 (-10072.0009, -10029.4955) -> (-10072.0826, -10029.534) ccw
  line L660 (-10072.0841, -10029.5794) -> (-10072.0826, -10029.534)
  ellipse E551 centre (-10071.975, -10009.5083) end of major axis (-10072.0743, -10009.5208) minor radius 0.0505 (-10072.0646, -10009.4946) -> (-10072.0744, -10009.5195) ccw
  line L661 (-10072.0744, -10009.5195) -> (-10072.0701, -10009.5759)
  line L662 (-10070.2098, -10008.8726) -> (-10070.2009, -10009.0284)
  line L663 (-10070.1977, -10008.9037) -> (-10070.2012, -10008.8419)
  ellipse E552 centre (-10070.4742, -10008.5856) end of major axis (-10070.7102, -10008.5029) minor radius 0.2103 (-10070.4216, -10008.7994) -> (-10070.4066, -10008.7975) ccw
  ellipse E553 centre (-10070.4742, -10008.5856) end of major axis (-10070.7102, -10008.5029) minor radius 0.2103 (-10070.5179, -10008.7919) -> (-10070.4895, -10008.7975) ccw
  ellipse E554 centre (-10072.0533, -10008.5057) end of major axis (-10072.2893, -10008.423) minor radius 0.2103 (-10072.097, -10008.712) -> (-10071.9857, -10008.7177) ccw
  spline S30 degree 3 poles (-10070.6584, -10008.4621) (-10070.6609, -10008.4654) (-10070.6659, -10008.4721) (-10070.6725, -10008.4826) (-10070.6783, -10008.4936) (-10070.6833, -10008.5049) (-10070.6874, -10008.5165) (-10070.6906, -10008.5285) (-10070.6928, -10008.5408) (-10070.694, -10008.5534) (-10070.6942, -10008.5663) (-10070.6933, -10008.5794) (-10070.6914, -10008.5928) (-10070.6883, -10008.6061) (-10070.6842, -10008.6193) (-10070.6791, -10008.6321) (-10070.6731, -10008.6446) (-10070.6684, -10008.6526) (-10070.6661, -10008.6565) knots 0 0 0 0 0.060272 0.120085 0.179563 0.238863 0.298168 0.35769 0.417672 0.478383 0.540118 0.603193 0.66794 0.734231 0.800525 0.866826 0.93328 1 1 1 1
  spline S31 degree 3 poles (-10070.5534, -10008.7516) (-10070.5498, -10008.7531) (-10070.5426, -10008.7561) (-10070.5315, -10008.76) (-10070.5203, -10008.7635) (-10070.5127, -10008.7654) (-10070.5089, -10008.7664) knots 0 0 0 0 0.249453 0.499322 0.749525 1 1 1 1
  spline S32 degree 3 poles (-10070.5179, -10008.7919) (-10070.521, -10008.791) (-10070.5272, -10008.7892) (-10070.5364, -10008.786) (-10070.5454, -10008.7823) (-10070.5543, -10008.7782) (-10070.563, -10008.7737) (-10070.5716, -10008.7688) (-10070.5799, -10008.7635) (-10070.5853, -10008.7597) (-10070.588, -10008.7578) knots 0 0 0 0 0.124037 0.24816 0.37249 0.497125 0.622143 0.747603 0.873547 1 1 1 1
  spline S33 degree 3 poles (-10070.6592, -10008.6806) (-10070.6619, -10008.6761) (-10070.6673, -10008.6671) (-10070.6745, -10008.6531) (-10070.6809, -10008.6388) (-10070.6866, -10008.6241) (-10070.6913, -10008.6093) (-10070.6953, -10008.5942) (-10070.6983, -10008.579) (-10070.7003, -10008.5638) (-10070.7014, -10008.5485) (-10070.7015, -10008.5333) (-10070.7005, -10008.5181) (-10070.6985, -10008.5031) (-10070.6953, -10008.4883) (-10070.691, -10008.4738) (-10070.6857, -10008.4598) (-10070.6813, -10008.4509) (-10070.6791, -10008.4465) knots 0 0 0 0 0.06406 0.128101 0.192047 0.25583 0.319386 0.382665 0.44563 0.508261 0.570562 0.63256 0.694313 0.755909 0.817476 0.879176 0.940214 1 1 1 1
  spline S34 degree 3 poles (-10070.2213, -10008.4589) (-10070.2199, -10008.4633) (-10070.2172, -10008.4722) (-10070.2143, -10008.486) (-10070.2121, -10008.5002) (-10070.2107, -10008.5149) (-10070.2102, -10008.5299) (-10070.2106, -10008.5453) (-10070.2118, -10008.561) (-10070.214, -10008.577) (-10070.2171, -10008.5933) (-10070.221, -10008.6097) (-10070.2258, -10008.6259) (-10070.2315, -10008.6417) (-10070.2379, -10008.657) (-10070.2452, -10008.6717) (-10070.2531, -10008.6859) (-10070.259, -10008.6949) (-10070.2619, -10008.6993) knots 0 0 0 0 0.054976 0.110963 0.168068 0.226392 0.286031 0.347076 0.409614 0.473728 0.539499 0.606943 0.674365 0.741 0.806864 0.871974 0.936347 1 1 1 1
  spline S35 degree 3 poles (-10070.3316, -10008.7681) (-10070.3345, -10008.7699) (-10070.3403, -10008.7734) (-10070.3492, -10008.7783) (-10070.3583, -10008.7827) (-10070.3676, -10008.7866) (-10070.3771, -10008.7901) (-10070.3867, -10008.7931) (-10070.3966, -10008.7956) (-10070.4032, -10008.7969) (-10070.4066, -10008.7975) knots 0 0 0 0 0.125299 0.25024 0.374942 0.499537 0.624172 0.749009 0.874221 1 1 1 1
  spline S36 degree 3 poles (-10070.3976, -10008.772) (-10070.3957, -10008.7717) (-10070.3918, -10008.7711) (-10070.386, -10008.77) (-10070.3803, -10008.7688) (-10070.3747, -10008.7674) (-10070.3691, -10008.7659) (-10070.3636, -10008.7641) (-10070.3582, -10008.7623) (-10070.3546, -10008.7609) (-10070.3528, -10008.7603) knots 0 0 0 0 0.12683 0.253009 0.378607 0.503687 0.628312 0.752538 0.876418 1 1 1 1
  spline S37 degree 3 poles (-10070.2127, -10008.4778) (-10070.2134, -10008.4761) (-10070.2149, -10008.4726) (-10070.2173, -10008.4675) (-10070.2198, -10008.4626) (-10070.2217, -10008.4594) (-10070.2227, -10008.4578) knots 0 0 0 0 0.252829 0.503515 0.752446 1 1 1 1
  spline S38 degree 3 poles (-10072.2692, -10008.447) (-10072.2698, -10008.4502) (-10072.2712, -10008.4564) (-10072.2725, -10008.466) (-10072.2732, -10008.4758) (-10072.2733, -10008.4857) (-10072.2728, -10008.4957) (-10072.2716, -10008.5059) (-10072.2697, -10008.5162) (-10072.2673, -10008.5265) (-10072.2642, -10008.5366) (-10072.2605, -10008.5466) (-10072.2563, -10008.5564) (-10072.2515, -10008.5659) (-10072.2462, -10008.5752) (-10072.2404, -10008.5842) (-10072.2342, -10008.593) (-10072.2297, -10008.5986) (-10072.2274, -10008.6014) knots 0 0 0 0 0.057782 0.11603 0.174905 0.234579 0.295234 0.357058 0.420245 0.484367 0.548389 0.61239 0.67646 0.740675 0.805095 0.869768 0.934728 1 1 1 1
  spline S39 degree 3 poles (-10072.097, -10008.712) (-10072.0981, -10008.7117) (-10072.1003, -10008.7111) (-10072.1036, -10008.7101) (-10072.1069, -10008.7091) (-10072.1091, -10008.7083) (-10072.1102, -10008.708) knots 0 0 0 0 0.249966 0.499931 0.749931 1 1 1 1
  spline S40 degree 3 poles (-10072.2209, -10008.6256) (-10072.2259, -10008.6189) (-10072.2357, -10008.6056) (-10072.2482, -10008.5842) (-10072.259, -10008.5618) (-10072.2678, -10008.5387) (-10072.2745, -10008.515) (-10072.2781, -10008.4949) (-10072.2798, -10008.4788) (-10072.2805, -10008.4668) (-10072.2806, -10008.4547) (-10072.2801, -10008.4467) (-10072.2798, -10008.4427) knots 0 0 0 0 0.126262 0.252787 0.379198 0.50514 0.630313 0.754513 0.81624 0.877714 0.938955 1 1 1 1
  spline S41 degree 3 poles (-10071.7895, -10008.4452) (-10071.7896, -10008.4537) (-10071.7896, -10008.4664) (-10071.7913, -10008.4836) (-10071.7931, -10008.4967) (-10071.7955, -10008.5101) (-10071.7996, -10008.5281) (-10071.8061, -10008.5502) (-10071.8161, -10008.5757) (-10071.8283, -10008.5998) (-10071.84, -10008.6185) (-10071.8503, -10008.6326) (-10071.8558, -10008.6392) (-10071.8586, -10008.6425) knots 0 0 0 0 0.118368 0.179357 0.241611 0.305185 0.370129 0.500874 0.629162 0.755042 0.878604 0.939568 1 1 1 1
  spline S42 degree 3 poles (-10071.9666, -10008.7134) (-10071.9682, -10008.7138) (-10071.9713, -10008.7146) (-10071.9761, -10008.7158) (-10071.9808, -10008.7168) (-10071.9841, -10008.7174) (-10071.9857, -10008.7177) knots 0 0 0 0 0.249221 0.498902 0.749131 1 1 1 1
  ellipse E555 centre (-10070.4653, -10008.5601) end of major axis (-10070.2294, -10008.6428) minor radius 0.2103 (-10070.5089, -10008.7664) -> (-10070.474, -10008.7729) ccw
  ellipse E556 centre (-10070.4653, -10008.5601) end of major axis (-10070.2294, -10008.6428) minor radius 0.2103 (-10070.4191, -10008.7744) -> (-10070.3976, -10008.772) ccw
  ellipse E557 centre (-10070.1532, -10008.6348) end of major axis (-10070.1386, -10008.3472) minor radius 0.0515 (-10070.2063, -10008.7407) -> (-10070.2047, -10008.7803) ccw
  ellipse E558 centre (-10070.1532, -10008.6348) end of major axis (-10070.1386, -10008.3472) minor radius 0.0515 (-10070.1855, -10008.4598) -> (-10070.2061, -10008.6733) ccw
  ellipse E559 centre (-10070.1532, -10008.6348) end of major axis (-10070.1702, -10008.9724) minor radius 0.0604 (-10070.1954, -10008.4541) -> (-10070.2157, -10008.7028) ccw
  ellipse E560 centre (-10070.1532, -10008.6348) end of major axis (-10070.1702, -10008.9724) minor radius 0.0604 (-10070.2151, -10008.7739) -> (-10070.2137, -10008.805) ccw
  ellipse E561 centre (-10072.2295, -10008.5299) end of major axis (-10072.2466, -10008.8674) minor radius 0.0604 (-10072.2838, -10008.4439) -> (-10072.292, -10008.6451) ccw
  line L664 (-10070.21, -10007.4565) -> (-10070.1033, -10007.1522)
  line L665 (-10070.1837, -10007.0962) -> (-10071.3727, -10007.0361)
  line L666 (-10071.4888, -10007.0821) -> (-10071.5955, -10007.3864)
  line L667 (-10070.1009, -10007.1951) -> (-10070.1928, -10007.4574)
  ellipse E562 centre (-10070.2016, -10007.1472) end of major axis (-10070.1018, -10007.1415) minor radius 0.051 (-10070.1033, -10007.1522) -> (-10070.1837, -10007.0962) ccw
  ellipse E563 centre (-10071.3906, -10007.0871) end of major axis (-10071.4904, -10007.0928) minor radius 0.051 (-10071.3727, -10007.0361) -> (-10071.4888, -10007.0821) ccw
  ellipse E564 centre (-10070.1991, -10007.1901) end of major axis (-10070.0993, -10007.1844) minor radius 0.051 (-10070.1009, -10007.1951) -> (-10070.0993, -10007.1844) ccw
  line L668 (-10070.1018, -10007.1415) -> (-10070.0993, -10007.1844)
  line L669 (-10070.2178, -10029.3835) -> (-10070.2028, -10029.4298)
  line L670 (-10072.2507, -10029.5635) -> (-10072.3044, -10029.3972)
  line L671 (-10070.2146, -10029.3387) -> (-10070.2006, -10029.382)
  line L672 (-10070.2178, -10029.3835) -> (-10070.318, -10029.3841)
  ellipse E565 centre (-10070.3539, -10029.2729) end of major axis (-10070.6033, -10029.255) minor radius 0.1101 (-10070.6008, -10029.2745) -> (-10070.318, -10029.3841) ccw
  line L673 (-10070.6008, -10029.2745) -> (-10070.7294, -10028.8766)
  line L674 (-10070.8425, -10028.8328) -> (-10072.0374, -10028.8406)
  line L675 (-10072.1218, -10028.8858) -> (-10072.0243, -10029.1876)
  ellipse E566 centre (-10072.2401, -10029.2854) end of major axis (-10072.4895, -10029.2675) minor radius 0.1101 (-10072.2042, -10029.3966) -> (-10072.0644, -10029.3738) ccw
  line L676 (-10072.2042, -10029.3966) -> (-10072.3044, -10029.3972)
  line L677 (-10072.0342, -10028.7958) -> (-10070.8393, -10028.788)
  line L678 (-10072.3012, -10029.3524) -> (-10072.201, -10029.3518)
  ellipse E567 centre (-10072.2369, -10029.2406) end of major axis (-10071.9876, -10029.2584) minor radius 0.1101 (-10072.201, -10029.3518) -> (-10072.0804, -10029.3355) ccw
  line L679 (-10070.7261, -10028.8318) -> (-10070.5976, -10029.2298)
  ellipse E568 centre (-10070.3507, -10029.2281) end of major axis (-10070.6001, -10029.2103) minor radius 0.1101 (-10070.5976, -10029.2298) -> (-10070.3148, -10029.3394) ccw
  line L680 (-10070.3148, -10029.3394) -> (-10070.2146, -10029.3387)
  line L681 (-10072.3044, -10029.3972) -> (-10072.3012, -10029.3524)
  line L682 (-10070.2146, -10029.3387) -> (-10070.2178, -10029.3835)
  ellipse E569 centre (-10070.8281, -10028.8772) end of major axis (-10070.7284, -10028.8844) minor radius 0.044 (-10070.7294, -10028.8766) -> (-10070.8425, -10028.8328) ccw
  ellipse E570 centre (-10072.023, -10028.8851) end of major axis (-10072.1228, -10028.878) minor radius 0.044 (-10072.0374, -10028.8406) -> (-10072.1218, -10028.8858) ccw
  ellipse E571 centre (-10070.8249, -10028.8325) end of major axis (-10070.7252, -10028.8396) minor radius 0.044 (-10070.7261, -10028.8318) -> (-10070.8393, -10028.788) ccw
  ellipse E572 centre (-10072.0198, -10028.8403) end of major axis (-10072.1196, -10028.8332) minor radius 0.044 (-10072.0342, -10028.7958) -> (-10072.1196, -10028.8332) ccw
  line L683 (-10072.1228, -10028.878) -> (-10072.1196, -10028.8332)
  line L684 (-10070.2557, -10009.3595) -> (-10070.2533, -10009.3874)
  line L685 (-10072.3423, -10009.3457) -> (-10072.325, -10009.5537)
  line L686 (-10070.2445, -10009.3841) -> (-10070.2487, -10009.3347)
  ellipse E573 centre (-10070.5231, -10009.1464) end of major axis (-10070.7638, -10009.0787) minor radius 0.2142 (-10070.5614, -10009.3575) -> (-10070.4496, -10009.3582) ccw
  ellipse E574 centre (-10072.1101, -10009.136) end of major axis (-10072.3508, -10009.0682) minor radius 0.2142 (-10072.1484, -10009.347) -> (-10072.0365, -10009.3477) ccw
  spline S43 degree 3 poles (-10070.5353, -10008.9397) (-10070.5489, -10008.9416) (-10070.5757, -10008.9453) (-10070.6139, -10008.9577) (-10070.6489, -10008.9744) (-10070.68, -10008.9955) (-10070.7063, -10009.0206) (-10070.727, -10009.0492) (-10070.739, -10009.0757) (-10070.7449, -10009.098) (-10070.7475, -10009.1153) (-10070.748, -10009.1331) (-10070.7465, -10009.1515) (-10070.7427, -10009.17) (-10070.7369, -10009.1885) (-10070.7291, -10009.2063) (-10070.7164, -10009.2292) (-10070.6962, -10009.2555) (-10070.6665, -10009.2829) (-10070.6324, -10009.3053) (-10070.5948, -10009.3228) (-10070.5679, -10009.3294) (-10070.5544, -10009.3326) knots 0 0 0 0 0.067054 0.132171 0.195214 0.256087 0.314845 0.371833 0.427831 0.455897 0.484265 0.513193 0.542966 0.573892 0.605563 0.637232 0.669027 0.733247 0.798614 0.865047 0.932273 1 1 1 1
  spline S44 degree 3 poles (-10070.5614, -10009.3575) (-10070.5682, -10009.3557) (-10070.5819, -10009.3522) (-10070.6081, -10009.3415) (-10070.6392, -10009.3234) (-10070.6724, -10009.2952) (-10070.7011, -10009.2618) (-10070.7246, -10009.2243) (-10070.7421, -10009.1838) (-10070.753, -10009.1416) (-10070.7558, -10009.1057) (-10070.7538, -10009.0774) (-10070.7502, -10009.0566) (-10070.7443, -10009.0366) (-10070.7365, -10009.0177) (-10070.7267, -10009.0001) (-10070.7116, -10008.9787) (-10070.6886, -10008.9551) (-10070.656, -10008.9324) (-10070.6194, -10008.915) (-10070.5801, -10008.9025) (-10070.5527, -10008.8984) (-10070.5389, -10008.8963) knots 0 0 0 0 0.031337 0.062781 0.126297 0.190936 0.256459 0.32232 0.387875 0.452577 0.516183 0.547678 0.57907 0.610325 0.640706 0.670386 0.69965 0.757762 0.816478 0.876441 0.937726 1 1 1 1
  spline S45 degree 3 poles (-10070.4266, -10008.897) (-10070.4142, -10008.8994) (-10070.3899, -10008.904) (-10070.3565, -10008.9189) (-10070.3275, -10008.9389) (-10070.3034, -10008.9642) (-10070.2844, -10008.994) (-10070.2709, -10009.0278) (-10070.2632, -10009.0653) (-10070.2616, -10009.1058) (-10070.2664, -10009.1484) (-10070.2773, -10009.1911) (-10070.2943, -10009.2318) (-10070.3167, -10009.2685) (-10070.3439, -10009.3004) (-10070.3703, -10009.3225) (-10070.3932, -10009.3369) (-10070.4112, -10009.3459) (-10070.43, -10009.3533) (-10070.443, -10009.3566) (-10070.4496, -10009.3582) knots 0 0 0 0 0.060227 0.117303 0.172542 0.227241 0.282631 0.339845 0.399897 0.463695 0.532058 0.603464 0.673189 0.741116 0.807351 0.872143 0.90418 0.93608 0.967968 1 1 1 1
  spline S46 degree 3 poles (-10070.4426, -10009.3334) (-10070.4393, -10009.3327) (-10070.4327, -10009.3314) (-10070.423, -10009.3288) (-10070.4135, -10009.3257) (-10070.4012, -10009.3211) (-10070.3863, -10009.3142) (-10070.3692, -10009.3044) (-10070.3531, -10009.2932) (-10070.3381, -10009.2806) (-10070.3241, -10009.267) (-10070.3156, -10009.257) (-10070.3114, -10009.252) knots 0 0 0 0 0.06406 0.127639 0.190828 0.253706 0.37877 0.503307 0.627605 0.751814 0.875967 1 1 1 1
  spline S47 degree 3 poles (-10070.266, -10009.0386) (-10070.2675, -10009.035) (-10070.2705, -10009.028) (-10070.2762, -10009.018) (-10070.2826, -10009.0087) (-10070.2897, -10008.9999) (-10070.2976, -10008.9918) (-10070.3061, -10008.9842) (-10070.3153, -10008.9773) (-10070.3251, -10008.9709) (-10070.3355, -10008.9652) (-10070.3465, -10008.96) (-10070.3581, -10008.9553) (-10070.3701, -10008.9512) (-10070.3827, -10008.9477) (-10070.3957, -10008.9447) (-10070.4092, -10008.9422) (-10070.4184, -10008.941) (-10070.423, -10008.9404) knots 0 0 0 0 0.059633 0.118254 0.176262 0.234034 0.291919 0.350232 0.409251 0.469215 0.530325 0.592744 0.656603 0.721998 0.789001 0.857656 0.927988 1 1 1 1